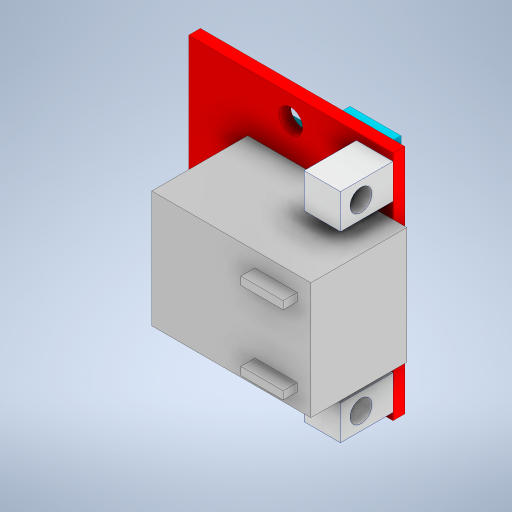
# Autodesk Inventor part: EGPL-T101-C1_DB
Saved by Autodesk Inventor 2024 (Build 280153000, 153)
## iProperties
Created: 2024-03-06
Part Number: EGPL-T101-C1_DB
Material: Generic
Document SubType Name: Modeling
Designer: Viktor
Density: 1 g/cm^3
Appearance: Default
Author: Viktor
Autodesk Inventor part; units mm, degrees
ref_plane "YZ Plane" through (0, 0, 0) normal (1, 0, 0) x (0, 1, 0)
ref_plane "XZ Plane" through (0, 0, 0) normal (0, 1, 0) x (-1, 0, 0)
ref_plane "XY Plane" through (0, 0, 0) normal (0, 0, 1) x (1, 0, 0)
sketch "Sketch1" plane through (0, 0, 0) normal (0, 0, 1) x (1, 0, 0)
  line L0 (-14, -15.875) -> (14, -15.875)
  line L1 (14, -15.875) -> (14, 15.875)
  line L2 (14, 15.875) -> (-14, 15.875)
  line L3 (-14, 15.875) -> (-14, -15.875)
  line L4 (-14, -15.875) -> (14, 15.875) construction
  line L5 (14, -15.875) -> (-14, 15.875) construction
  line L6 (0, 22.225) -> (0, -22.225) construction
  circle A0 centre (0, 12.7) radius 1.63
  line L7 (-19.6, 0) -> (19.6, 0) construction
  circle A1 centre (0, -12.7) radius 1.63
  point P0 (0, 0)
  dimension "d0" = 28
  dimension "d1" = 31.75
  dimension "d2" = 25.4
  dimension "d3" = 3.26
  constraints: 12 end point, 2 centre point, 2 midpoint, 2 parallel, 1 horizontal, 1 perpendicular, 1 point on line, 1 symmetric about line, 1 other
  measures "d0" distance of L1.end L2.end
  measures "d1" distance of L0.end L1.end
  measures "d2" distance of A1.centre A0.centre
  measures "d3" diameter of A0
extrude "Extrusion1" add sketch "Sketch1" along normal blind 1.6
sketch "Sketch2" plane through (0, 0, 1.6) normal (0, 0, 1) x (1, 0, 0)
  line L0 (-19.978, 0) -> (21.868, 0) projected
  line L1 (-5.91, 8) -> (15.89, 8)
  line L2 (15.89, 8) -> (15.89, -8)
  line L3 (15.89, -8) -> (-5.91, -8)
  line L4 (-5.91, -8) -> (-5.91, 8)
  line L5 (-5.91, 8) -> (15.89, -8) construction
  line L6 (15.89, 8) -> (-5.91, -8) construction
  line L7 (14, -15.875) -> (14, 15.875) projected
  point P0 (0, 0)
  point P1 (4.99, 0)
  point P2 (14, -8)
  point P3 (14, 8)
  dimension "d6" = 16
  dimension "d7" = 21.8
  dimension "d8" = 1.89
  constraints: 12 end point, 2 midpoint, 2 parallel, 1 horizontal, 1 perpendicular, 1 point on line
  measures "d6" distance of L1.end L2.end
  measures "d7" distance of L2.end L3.end
  measures "d8" distance between parallel lines of L7 L2
extrude "Extrusion2" add sketch "Sketch2" along normal blind 13.15 separate body
sketch "Sketch3" plane through (0, 0, 14.75) normal (0, 0, 1) x (1, 0, 0)
  line L0 (14, 8) -> (-5.91, 8) projected
  line L1 (-5.91, 8) -> (-5.91, -8) projected
  line L2 (-5.91, -8) -> (14, -8) projected
  line L3 (14, -8) -> (14, 8) projected
  line L4 (14, -4.8) -> (8.2, -4.8)
  line L5 (8.2, -4.8) -> (8.2, -5.9)
  line L6 (8.2, -5.9) -> (14, -5.9)
  line L7 (14, -5.9) -> (14, -4.8)
  line L8 (-19.978, 0) -> (21.868, 0) projected
  line L9 (14, 4.8) -> (8.2, 4.8)
  line L10 (8.2, 4.8) -> (8.2, 5.9)
  line L11 (8.2, 5.9) -> (14, 5.9)
  line L12 (14, 5.9) -> (14, 4.8)
  point P0 (0, 0)
  dimension "d11" = 5.8
  dimension "d12" = 3.2
  dimension "d13" = 1.1
  constraints: 16 end point, 4 symmetric about line, 2 parallel, 1 horizontal, 1 perpendicular, 1 point on line
  measures "d11" distance of L5.end L6.end
  measures "d12" distance between parallel lines of L2 L4
  measures "d13" distance of L4.end L5.end
extrude "Extrusion3" add sketch "Sketch3" along normal blind 1.9 contours L3 L9 L10 L11 | L3 L6 L5 L4 bodies 2
sketch "Sketch4" plane through (0, 0, 1.6) normal (0, 0, 1) x (1, 0, 0)
  circle A0 centre (0, -12.7) radius 1.63 projected
  circle A1 centre (0, 12.7) radius 1.63 projected
  line L0 (14, -15.875) -> (14, 15.875) projected
  line L1 (14, 15.875) -> (-14, 15.875) projected
  line L2 (-14, 15.875) -> (-14, -15.875) projected
  line L3 (-14, -15.875) -> (14, -15.875) projected
  line L4 (14, -14.9) -> (9, -14.9)
  line L5 (9, -14.9) -> (9, -10.15)
  line L6 (9, -10.15) -> (14, -10.15)
  line L7 (14, -10.15) -> (14, -14.9)
  line L8 (-19.6, 0) -> (19.6, 0) projected
  line L9 (14, 14.9) -> (9, 14.9)
  line L10 (9, 14.9) -> (9, 10.15)
  line L11 (9, 10.15) -> (14, 10.15)
  line L12 (14, 10.15) -> (14, 14.9)
  point P0 (0, 0)
  point P1 (14, 12.525)
  point P2 (14, -12.525)
  dimension "d16" = 4.75
  dimension "d18" = 25.05
  constraints: 16 end point, 4 symmetric about line, 2 midpoint, 2 parallel, 1 horizontal, 1 perpendicular
  measures "d16" distance between parallel lines of L6 L4
  measures "d18" distance of point (14, 12.525) point (14, -12.525)
extrude "Extrusion4" add sketch "Sketch4" along normal blind 7.2 separate body contours L4 L5 L6 L0 | L11 L10 L9 L0
sketch "Sketch5" plane through (14, -15.875, 0) normal (1, 0, 0) x (0, 0, -1)
  line L0 (-8.8, 3.35) -> (-3.1193, 3.35) construction
  line L1 (-19.98, 15.875) -> (3.33, 15.875) projected
  circle A0 centre (-6, 3.35) radius 1.5
  line L2 (-1.6, 0) -> (-1.6, 31.75) projected
  circle A1 centre (-6, 28.4) radius 1.5
  line L3 (-8.8, 0.975) -> (-8.8, 5.725) projected
  point P0 (0, 15.875)
  point P1 (-1.6, 5.725)
  point P2 (-1.6, 7.875)
  point P3 (-1.6, 26.025)
  dimension "d21" = 3
  dimension "d22" = 4.4
  constraints: 2 centre point, 2 end point, 1 horizontal, 1 midpoint, 1 point on line, 1 symmetric about line, 1 other
  measures "d21" diameter of A0
  measures "d22" distance from line of L2 A0.centre
extrude "Extrusion5" cut sketch "Sketch5" against normal blind 7.2 bodies 3
sketch "Sketch6" plane through (0, 0, 0) normal (0, 0, -1) x (-1, 0, 0)
  line L0 (-19.6, 0) -> (19.6, 0) construction
  line L1 (7.7, 7.65) -> (10.7, 7.65)
  line L2 (10.7, 7.65) -> (10.7, -7.65)
  line L3 (10.7, -7.65) -> (7.7, -7.65)
  line L4 (7.7, -7.65) -> (7.7, 7.65)
  line L5 (7.7, 7.65) -> (10.7, -7.65) construction
  line L6 (10.7, 7.65) -> (7.7, -7.65) construction
  line L7 (14, 15.875) -> (14, -15.875) projected
  point P0 (0, 0)
  point P1 (9.2, 0)
  dimension "d25" = 15.3
  dimension "d26" = 3
  dimension "d27" = 3.3
  constraints: 12 end point, 2 midpoint, 2 parallel, 1 horizontal, 1 perpendicular, 1 point on line
  measures "d25" distance of L1.end L2.end
  measures "d26" distance between parallel lines of L4 L2
  measures "d27" distance between parallel lines of L7 L2
extrude "Extrusion6" add sketch "Sketch6" along normal blind 2 separate body
sketch "Sketch7" plane through (0, 0, 0) normal (0, 0, -1) x (-1, 0, 0)
  line L0 (-19.6, 0) -> (19.6, 0) construction
  line L1 (6.5, 9.875) -> (-11.5, 9.875)
  line L2 (-11.5, 9.875) -> (-11.5, -9.875)
  line L3 (-11.5, -9.875) -> (6.5, -9.875)
  line L4 (6.5, -9.875) -> (6.5, 9.875)
  line L5 (6.5, 9.875) -> (-11.5, -9.875) construction
  line L6 (-11.5, 9.875) -> (6.5, -9.875) construction
  line L7 (-4.5, -9.875) -> (-11.5, -9.875)
  line L8 (-11.5, -9.875) -> (-11.5, -14.875)
  line L9 (-11.5, -14.875) -> (-4.5, -14.875)
  line L10 (-4.5, -14.875) -> (-4.5, -9.875)
  line L11 (-4.5, 9.875) -> (-11.5, 9.875)
  line L12 (-11.5, 9.875) -> (-11.5, 14.875)
  line L13 (-11.5, 14.875) -> (-4.5, 14.875)
  line L14 (-4.5, 14.875) -> (-4.5, 9.875)
  line L15 (14, -15.875) -> (-14, -15.875) projected
  line L16 (-14, -15.875) -> (-14, 15.875) projected
  point P0 (0, 0)
  point P1 (-2.5, 0)
  point P2 (-11.5, 9.875)
  dimension "d30" = 1
  dimension "d31" = 2.5
  dimension "d32" = 2.5
  dimension "d33" = 5
  dimension "d34" = 7
  dimension "d35" = 18
  constraints: 28 end point, 5 symmetric about line, 4 parallel, 2 horizontal, 2 midpoint, 2 perpendicular, 2 point on line
  measures "d30" distance between parallel lines of L15 L9
  measures "d31" distance between parallel lines of L16 L8
  measures "d32" distance between parallel lines of L16 L2
  measures "d33" distance between parallel lines of L9 L7
  measures "d34" distance between parallel lines of L8 L10
  measures "d35" distance between parallel lines of L2 L4
extrude "Extrusion7" add sketch "Sketch7" along normal blind 2 separate body
equation "\"d32\" = d31"
body "Solid1"
body "Solid2"
body "Solid3"
body "Solid4"
body "Solid5"
